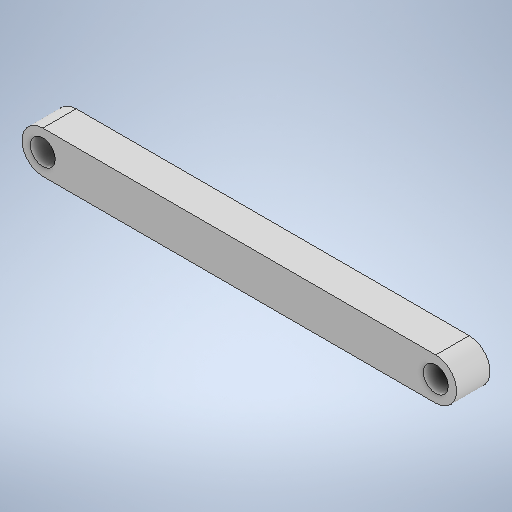
# Autodesk Inventor part: SteeringAxis
Saved by Autodesk Inventor 2025.2 (Build 292293000, 293)
## iProperties
Created: 2025-01-08
Part Number: SteeringAxis
Material: 일반
Document SubType Name: Modeling
Designer: SEON
Density: 1 g/cm^3
Appearance: 기본값
Author: SEON
Autodesk Inventor part; units mm, degrees
ref_plane "YZ Plane" through (0, 0, 0) normal (1, 0, 0) x (0, 1, 0)
ref_plane "XZ Plane" through (0, 0, 0) normal (0, 1, 0) x (-1, 0, 0)
ref_plane "XY Plane" through (0, 0, 0) normal (0, 0, 1) x (1, 0, 0)
sketch "스케치1" plane through (0, 0, 0) normal (0, 0, 1) x (1, 0, 0)
  line L0 (0, 0) -> (47.013, 0) construction
  line L1 (0, -2.5) -> (47.013, -2.5)
  line L2 (47.013, 2.5) -> (0, 2.5)
  arc A0 (0, 2.5) -> (0, -2.5) centre (0, 0) ccw
  arc A1 (47.013, -2.5) -> (47.013, 2.5) centre (47.013, 0) ccw
  circle A2 centre (0, 0) radius 1.5
  circle A3 centre (47.013, 0) radius 1.5
  point P0 (23.5065, 0)
  point P1 (49.513, 0)
  point P2 (-2.5, 0)
  dimension "d0" = 5
  dimension "d4" = 3
  dimension "d5" = 3
  dimension "d6" = 47.013
  constraints: 8 end point, 6 point on circle, 4 centre point, 4 tangent, 2 coincident, 1 horizontal, 1 midpoint, 1 parallel
  measures "d0" diameter of A1
  measures "d4" diameter of A2
  measures "d5" diameter of A3
  measures "d6" distance of L0.start L0.end
extrude "돌출1" add sketch "스케치1" along normal blind 4
